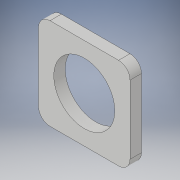
# Autodesk Inventor part: MotorBlock
Saved by Autodesk Inventor 2018 (Build 220112000, 112)
## iProperties
Created: 2020-03-23
Part Number: MotorBlock
Material: Generic
Document SubType Name: Modeling
Designer: emile
Density: 1 g/cm^3
Appearance: Default
Author: emile
Autodesk Inventor part; units mm, degrees
ref_plane "YZ Plane" through (0, 0, 0) normal (1, 0, 0) x (0, 1, 0)
ref_plane "XZ Plane" through (0, 0, 0) normal (0, 1, 0) x (-1, 0, 0)
ref_plane "XY Plane" through (0, 0, 0) normal (0, 0, 1) x (1, 0, 0)
sketch "Sketch1" plane through (0, 0, 0) normal (0, 0, 1) x (1, 0, 0)
  circle A0 centre (0, 0) radius 33.909
  line L0 (50.8, -50.8) -> (-50.8, -50.8)
  line L1 (-50.8, -50.8) -> (-50.8, 50.8)
  line L2 (-50.8, 50.8) -> (50.8, 50.8)
  line L3 (50.8, 50.8) -> (50.8, -50.8)
  line L4 (50.8, -50.8) -> (-50.8, 50.8) construction
  line L5 (-50.8, -50.8) -> (50.8, 50.8) construction
  dimension "d0" = 67.818
  dimension "d1" = 101.6
  dimension "d2" = 101.6
  constraints: 12 end point, 2 midpoint, 2 parallel, 1 centre point, 1 coincident, 1 horizontal, 1 perpendicular
  measures "d0" diameter of A0
  measures "d1" distance of L1.end L2.end
  measures "d2" distance of L2.end L0.start
extrude "Extrusion1" add sketch "Sketch1" along normal blind 12.7
fillet "Fillet1" radius 12.7 4 edges at (50.8, 50.8, 6.35) (50.8, -50.8, 6.35) (-50.8, 50.8, 6.35) (-50.8, -50.8, 6.35)
body "Solid1"
